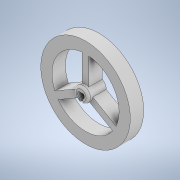
# Autodesk Inventor part: Колесо D40 под ось моторов серии N
Saved by Autodesk Inventor 2020 (Build 240168000, 168)
## iProperties
Created: 2021-03-15
Part Number: Колесо D40 под ось моторов серии N
Material: Типовые
Document SubType Name: Modeling
Designer: Антон
Density: 1 g/cm^3
Appearance: По умолчанию
Author: Антон
Autodesk Inventor part; units mm, degrees
ref_plane "YZ Plane" through (0, 0, 0) normal (1, 0, 0) x (0, 1, 0)
ref_plane "XZ Plane" through (0, 0, 0) normal (0, 1, 0) x (-1, 0, 0)
ref_plane "XY Plane" through (0, 0, 0) normal (0, 0, 1) x (1, 0, 0)
sketch "Эскиз1" plane through (0, 0, 0) normal (0, 0, 1) x (1, 0, 0)
  circle A0 centre (0, 0) radius 20
  circle A1 centre (0, 0) radius 15
  circle A2 centre (0, 0) radius 3.25
  line L0 (0, 15) -> (12.9904, -7.5)
  line L1 (12.9904, -7.5) -> (-12.9904, -7.5)
  line L2 (-12.9904, -7.5) -> (0, 15)
  line L3 (1.5, -15) -> (1.5, 15)
  line L4 (1.5, 15) -> (-1.5, 15)
  line L5 (-1.5, 15) -> (-1.5, -15)
  line L6 (-1.5, -15) -> (1.5, -15)
  line L7 (1.5, -15) -> (-1.5, 15) construction
  line L8 (1.5, 15) -> (-1.5, -15) construction
  line L9 (13.7404, 6.201) -> (-12.2404, -8.799)
  line L10 (-12.2404, -8.799) -> (-13.7404, -6.201)
  line L11 (-13.7404, -6.201) -> (12.2404, 8.799)
  line L12 (12.2404, 8.799) -> (13.7404, 6.201)
  line L13 (13.7404, 6.201) -> (-13.7404, -6.201) construction
  line L14 (-12.2404, -8.799) -> (12.2404, 8.799) construction
  line L15 (-13.7404, 6.201) -> (12.2404, -8.799)
  line L16 (12.2404, -8.799) -> (13.7404, -6.201)
  line L17 (13.7404, -6.201) -> (-12.2404, 8.799)
  line L18 (-12.2404, 8.799) -> (-13.7404, 6.201)
  line L19 (-13.7404, 6.201) -> (13.7404, -6.201) construction
  line L20 (12.2404, -8.799) -> (-12.2404, 8.799) construction
  point P0 (1.5, 14.9248)
  point P1 (13.6753, -6.1634)
  point P2 (3.2469, -0.1425)
  point P3 (1.5, 2.8831)
  point P4 (1.7469, -2.7406)
  point P5 (12.1753, -8.7614)
  point P6 (-12.1753, -8.7614)
  point P7 (-1.7469, -2.7406)
  point P8 (-1.5, 14.9248)
  point P9 (-1.5, 2.8831)
  point P10 (-3.2469, -0.1425)
  point P11 (-13.6753, -6.1634)
  dimension "d1" = 30
  dimension "d0" = 40
  dimension "d2" = 6.5
  dimension "d3" = 3
  dimension "d4" = 3
  dimension "d5" = 3
  constraints: 42 end point, 6 midpoint, 6 parallel, 4 coincident, 3 perpendicular, 2 centre point, 1 vertical, 10 other
  measures "d0" diameter of A0
  measures "d2" diameter of A2
  measures "d3" distance of L4.end L3.end
  measures "d4" distance of L9.end L10.end
  measures "d5" distance of L16.end L15.end
extrude "Выдавливание1" add sketch "Эскиз1" along normal blind 6 contours A0 | A1 L12 L9 | L17 L16 A1 | A1 L0 L17 | A1 L11 L12 | L16 L15 A1 | L1 L15 A2 L17 L0 | A1 L15 L1 | L9 L17 L3 L11 A2 | A2 L17 L9 | A2 L15 L3 L9 L17 | L3 L0 A1 | A1 L4 L3 | L3 A2 L5 L2 L0 | L11 L3 A2 | L9 L3 L17 | L3 L6 A1 | A2 L3 L15 | L2 L5 A1 | A1 L5 L4 | L3 L11 L17 L5 A2 | L3 L17 L11 | L9 L15 L5 L11 L17 L3 | L3 L15 L9 | L6 L5 A1 | A2 L5 L9 L15 L3 | L5 L17 A2 | L11 L5 L17 | L9 L5 L15 | L9 A1 L1 | L1 L2 L11 A2 L9 | A2 L9 L5 | A1 L18 L17 | L17 L5 L11 L15 A2 | L5 L15 L11 | L9 A2 L11 L15 L5 | L9 L10 A1 | L10 L11 A1 | A1 L11 L2 | A1 L15 L18 | L15 L11 A2
sketch "Эскиз2" plane through (0, 0, 6) normal (0, 0, 1) x (1, 0, 0)
  circle A0 centre (0, 0) radius 3.25
  constraints: 1 centre point, 1 coincident
extrude "Выдавливание2" add sketch "Эскиз2" along normal blind 2
sketch "Эскиз3" plane through (0, 0, 8) normal (0, 0, 1) x (1, 0, 0)
  circle A0 centre (0, 0) radius 1.5
  line L0 (-1.5, -1) -> (1.5, -1)
  line L1 (1.5, -1) -> (1.5, 1)
  line L2 (1.5, 1) -> (-1.5, 1)
  line L3 (-1.5, 1) -> (-1.5, -1)
  line L4 (-1.5, -1) -> (1.5, 1) construction
  line L5 (1.5, -1) -> (-1.5, 1) construction
  line L6 (0.75, 3.2651) -> (-0.75, 3.2651)
  line L7 (-0.75, 3.2651) -> (-0.75, -3.2651)
  line L8 (-0.75, -3.2651) -> (0.75, -3.2651)
  line L9 (0.75, -3.2651) -> (0.75, 3.2651)
  line L10 (0.75, 3.2651) -> (-0.75, -3.2651) construction
  line L11 (-0.75, 3.2651) -> (0.75, -3.2651) construction
  point P0 (-1.118, 1)
  point P1 (-0.75, -1.299)
  point P2 (0.75, -1.299)
  point P3 (1.118, 1)
  dimension "d10" = 3
  dimension "d11" = 2
  dimension "d12" = 1.5
  constraints: 24 end point, 4 midpoint, 4 parallel, 2 horizontal, 2 perpendicular, 1 centre point, 1 coincident
  measures "d10" diameter of A0
  measures "d11" distance of L1.end L0.end
  measures "d12" distance of L8.end L7.end
extrude "Выдавливание3" cut sketch "Эскиз3" against normal through all contours A0 L0 L9 L2 | A0 L9 L0 | L9 L0 L7 L2 | L9 L8 L7 A0 | A0 L7 L0 L9 | L7 L0 A0 L2 | A0 L0 L7
fillet "Сопряжение1" radius 1 1 edges at (-3.25, 0, 8)
